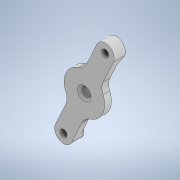
# Autodesk Inventor part: motor_pin_shell_1
Saved by Autodesk Inventor 2020 (Build 240168000, 168)
## iProperties
Created: 2021-02-22
Part Number: motor_pin_shell_1
Material: Generic
Document SubType Name: Modeling
Designer: Shuang Peng
Density: 1 g/cm^3
Appearance: Default
Author: Shuang Peng
Autodesk Inventor part; units mm, degrees
ref_plane "YZ Plane" through (0, 0, 0) normal (1, 0, 0) x (0, 1, 0)
ref_plane "XZ Plane" through (0, 0, 0) normal (0, 1, 0) x (-1, 0, 0)
sketch "Sketch1" plane through (0, 0, 0) normal (0, 0, 1) x (1, 0, 0)
  arc A0 (-3.1637, -10.5352) -> (9.2384, -5.9709) centre (0, 0) ccw projected
  arc A1 (-5.9709, -9.2384) -> (-3.1637, -10.5352) centre (-4.6131, -9.986) ccw projected
  arc A2 (-10.5352, 3.1637) -> (-5.9709, -9.2384) centre (0, 0) ccw projected
  arc A3 (-9.2384, 5.9709) -> (-10.5352, 3.1637) centre (-9.986, 4.6131) ccw projected
  arc A4 (3.1637, 10.5352) -> (-9.2384, 5.9709) centre (0, 0) ccw projected
  arc A5 (5.9709, 9.2384) -> (3.1637, 10.5352) centre (4.6131, 9.986) ccw projected
  arc A6 (10.5352, -3.1637) -> (5.9709, 9.2384) centre (0, 0) ccw projected
  arc A7 (9.2384, -5.9709) -> (10.5352, -3.1637) centre (9.986, -4.6131) ccw projected
  circle A8 centre (-19.9719, 9.2261) radius 1.55 projected
  circle A9 centre (19.9719, -9.2261) radius 1.55 projected
  circle A10 centre (-9.2261, -19.9719) radius 1.55 projected
  circle A11 centre (9.2261, 19.9719) radius 1.55 projected
  arc A12 (13.9995, -0.1171) -> (10.5836, 9.1644) centre (0, 0) ccw projected
  arc A13 (10.1281, 12.3863) -> (10.5836, 9.1644) centre (12.8516, 11.1282) ccw projected
  line L0 (10.1281, 12.3863) -> (12.8574, 18.2945) projected
  arc A14 (12.8574, 18.2945) -> (5.5949, 21.6494) centre (9.2261, 19.9719) ccw projected
  line L1 (5.5949, 21.6494) -> (2.8656, 15.7413) projected
  arc A15 (0.1171, 13.9995) -> (2.8656, 15.7413) centre (0.1422, 16.9994) ccw projected
  arc A16 (0.1171, 13.9995) -> (-9.1644, 10.5836) centre (0, 0) ccw projected
  arc A17 (-12.3863, 10.1281) -> (-9.1644, 10.5836) centre (-11.1282, 12.8516) ccw projected
  line L2 (-12.3863, 10.1281) -> (-18.2945, 12.8574) projected
  arc A18 (-18.2945, 12.8574) -> (-21.6494, 5.5949) centre (-19.9719, 9.2261) ccw projected
  line L3 (-21.6494, 5.5949) -> (-15.7413, 2.8656) projected
  arc A19 (-13.9995, 0.1171) -> (-15.7413, 2.8656) centre (-16.9994, 0.1422) ccw projected
  arc A20 (-13.9995, 0.1171) -> (-10.5836, -9.1644) centre (0, 0) ccw projected
  arc A21 (-10.1281, -12.3863) -> (-10.5836, -9.1644) centre (-12.8516, -11.1282) ccw projected
  line L4 (-10.1281, -12.3863) -> (-12.8574, -18.2945) projected
  arc A22 (-12.8574, -18.2945) -> (-5.5949, -21.6494) centre (-9.2261, -19.9719) ccw projected
  line L5 (-5.5949, -21.6494) -> (-2.8656, -15.7413) projected
  arc A23 (-0.1171, -13.9995) -> (-2.8656, -15.7413) centre (-0.1422, -16.9994) ccw projected
  arc A24 (-0.1171, -13.9995) -> (9.1644, -10.5836) centre (0, 0) ccw projected
  arc A25 (12.3863, -10.1281) -> (9.1644, -10.5836) centre (11.1282, -12.8516) ccw projected
  line L6 (12.3863, -10.1281) -> (18.2945, -12.8574) projected
  arc A26 (18.2945, -12.8574) -> (21.6494, -5.5949) centre (19.9719, -9.2261) ccw projected
  line L7 (21.6494, -5.5949) -> (15.7413, -2.8656) projected
  arc A27 (13.9995, -0.1171) -> (15.7413, -2.8656) centre (16.9994, -0.1422) ccw projected
  circle A28 centre (0, 0) radius 5.575 projected
  circle A29 centre (0, 0) radius 9 projected
  circle A30 centre (0, 0) radius 9
  line L8 (9.2261, 19.9719) -> (-9.2261, -19.9719) construction
  line L9 (5.5949, 21.6494) -> (-12.8574, -18.2945)
  line L10 (-5.5949, -21.6494) -> (12.8574, 18.2945)
  arc A31 (12.8574, 18.2945) -> (5.5949, 21.6494) centre (9.2261, 19.9719) ccw
  arc A32 (-12.8574, -18.2945) -> (-5.5949, -21.6494) centre (-9.2261, -19.9719) ccw
  point P0 (0, 0)
  point P1 (0, 0)
  point P2 (-0.2502, 8.9965)
  point P3 (-7.0123, -5.6416)
  point P4 (-10.1281, -12.3863)
  point P5 (0.2502, -8.9965)
  point P6 (7.0123, 5.6416)
  dimension "d0" = 18
  dimension "d1" = 8
  constraints: 8 end point, 4 point on circle, 4 tangent, 3 centre point, 1 coincident, 1 midpoint, 1 parallel
  measures "d0" diameter of A30
  measures "d1" diameter of A32
extrude "Extrusion1" add sketch "Sketch1" along normal blind 3 contours A1 A2 L9 A29 L10 A0 | A0 L10 L5 A22 L4 L9 A2 A1 | L10 A28 A29 | A29 L9 A28 L10 | A29 L9 A28 | L10 A28 | A28 L9 L10 | L10 A29 L9 A4 A5 A6 | A6 A5 A4 L9 L1 A14 L0 L10 | A29 L10 A28 L9 | A28 L9
fillet "Fillet1" radius 6 4 edges at (-7.0123, -5.6416, 1.5) (-0.2502, 8.9965, 1.5) (0.2502, -8.9965, 1.5) (7.0123, 5.6416, 1.5)
sketch "Sketch2" plane through (0, 0, 3) normal (0, 0, 1) x (1, 0, 0)
  circle A0 centre (0, 0) radius 5.575 projected
  circle A1 centre (0, 0) radius 2
  point P0 (0, 0)
  dimension "d5" = 4
  constraints: 1 centre point, 1 coincident
  measures "d5" diameter of A1
extrude "Extrusion2" cut sketch "Sketch2" against normal blind 3 contours A1
sketch "Sketch3" plane through (0, 0, 0) normal (0, 0, -1) x (-1, 0, 0)
  circle A0 centre (0, 0) radius 6.5 projected
  circle A1 centre (0, 0) radius 5.75 projected
  circle A2 centre (0, 0) radius 6
  circle A3 centre (0, 0) radius 5.5
  circle A4 centre (0, 0) radius 2
  point P0 (0, 0)
  dimension "d8" = 12
  dimension "d9" = 11
  dimension "d10" = 4
  constraints: 3 centre point, 3 coincident
  measures "d8" diameter of A2
  measures "d9" diameter of A3
  measures "d10" diameter of A4
extrude "Extrusion3" add sketch "Sketch3" along normal blind 1 contours A3
chamfer "Chamfer1" distance 1 angle 45 1 edges at (-2, 0, 3)
sketch "Sketch4" plane through (0, 0, 0) normal (0, 0, -1) x (-1, 0, 0)
  circle A0 centre (0, 0) radius 5.5 projected
  arc A1 (8.2601, -3.5736) -> (8.32, -8.4722) centre (13.7669, -5.956) ccw projected
  arc A2 (8.2601, -3.5736) -> (2.6337, 8.606) centre (0, 0) ccw projected
  arc A3 (-1.0574, 11.8272) -> (2.6337, 8.606) centre (4.3894, 14.3434) ccw projected
  line L0 (-5.5949, 21.6494) -> (-1.0574, 11.8272) projected
  arc A4 (-5.5949, 21.6494) -> (-12.8574, 18.2945) centre (-9.2261, 19.9719) ccw projected
  line L1 (-8.32, 8.4722) -> (-12.8574, 18.2945) projected
  arc A5 (-8.2601, 3.5736) -> (-8.32, 8.4722) centre (-13.7669, 5.956) ccw projected
  arc A6 (-8.2601, 3.5736) -> (-2.6337, -8.606) centre (0, 0) ccw projected
  arc A7 (1.0574, -11.8272) -> (-2.6337, -8.606) centre (-4.3894, -14.3434) ccw projected
  line L2 (5.5949, -21.6494) -> (1.0574, -11.8272) projected
  arc A8 (5.5949, -21.6494) -> (12.8574, -18.2945) centre (9.2261, -19.9719) ccw projected
  line L3 (8.32, -8.4722) -> (12.8574, -18.2945) projected
  circle A9 centre (-9.2261, 19.9719) radius 1.55 projected
  circle A10 centre (9.2261, -19.9719) radius 1.55 projected
  circle A11 centre (-9.2261, 19.9719) radius 4
  circle A12 centre (9.2261, -19.9719) radius 4
  point P0 (0, 0)
  point P1 (-12.8574, 18.2945)
  point P2 (12.8574, -18.2945)
  dimension "d16" = 8
  dimension "d17" = 8
  constraints: 2 centre point, 2 coincident
  measures "d16" diameter of A11
  measures "d17" diameter of A12
ref_plane "Work Plane1" through (-24.1436, -24.1436, -2) normal (0, 0, 1) x (1, 0, 0)
extrude "Extrusion4" add sketch "Sketch4" along normal up to surface (2 mm away) contours A8 A12 | A11 A4
fillet "Fillet2" radius 2 2 edges at (7.5487, 16.3407, 0) (-7.5487, -16.3407, 0)
chamfer "Chamfer2" distance 1 angle 45 1 edges at (5.5, 0, -1)
body "Solid1"
